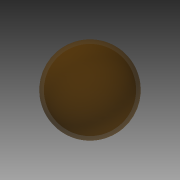
# Autodesk Inventor part: bodySphere
Saved by Autodesk Inventor 2013 (Build 170138000, 138)
## iProperties
Created: 2013-01-08
Part Number: bodySphere
Material: Polycarbonate, Clear
Document SubType Name: Modeling
Designer: Nano
Mass: 3408.07 g
Surface Area: 4479.29 cm^2
Volume: 2840.06 cm^3
Density: 1.2 g/cm^3
Author: Nano
Autodesk Inventor part; units mm, degrees
ref_plane "YZ Plane" through (0, 0, 0) normal (1, 0, 0) x (0, 1, 0)
ref_plane "XZ Plane" through (0, 0, 0) normal (0, 1, 0) x (-1, 0, 0)
ref_plane "XY Plane" through (0, 0, 0) normal (0, 0, 1) x (1, 0, 0)
sketch "Sketch1" plane through (0, 0, 0) normal (0, 0, 1) x (1, 0, 0)
  circle A0 centre (0, 0) radius 139.7
  line L0 (113.488448, 81.464484) -> (-113.488448, -81.464484)
  dimension "d0" = 279.4
  constraints: 2 end point, 2 point on circle, 1 centre point, 1 coincident, 1 midpoint
  measures "d0" diameter of A0
revolve "Revolution1" add sketch "Sketch1" angle 360 about axis through (113.488448, 81.464484, 0) along (-0.8123726, -0.5831388, 0) picked at (-24.909298, 39.344394) contours L0 A0
shell "Shell1" thickness 12.7 removed faces 0
body "Solid1"
